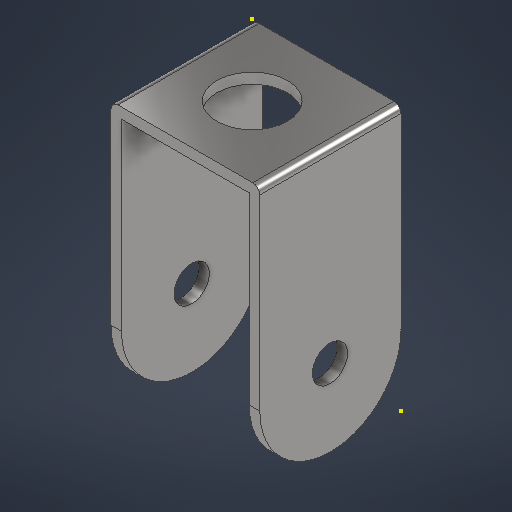
# Autodesk Inventor part: peca1
Saved by Autodesk Inventor 2026 (Build 300175050, 175E)
## iProperties
Created: 2026-05-07
Part Number: peca1
Material: Steel, Carbon
Document SubType Name: Modeling
Designer: Administrator
Density: 7.85 g/cm^3
Appearance: Semi-Polished
Mass: 155.634 g
Surface Area: 148.219 cm^2
Volume: 19.826 cm^3
Author: Administrator
Autodesk Inventor part; units mm, degrees
ref_plane "YZ Plane" through (0, 0, 0) normal (1, 0, 0) x (0, 1, 0)
ref_plane "XZ Plane" through (0, 0, 0) normal (0, 1, 0) x (-1, 0, 0)
ref_plane "XY Plane" through (0, 0, 0) normal (0, 0, 1) x (1, 0, 0)
sketch "Sketch1" plane through (0, 0, 0) normal (0, 0, 1) x (1, 0, 0)
  line L0 (0, 0) -> (3, 0)
  line L1 (3, 0) -> (3, 72)
  line L2 (3, 72) -> (39.1537, 72)
  line L3 (42.1537, 75) -> (0, 75)
  line L4 (0, 75) -> (0, 0)
  line L5 (42.1537, 75) -> (42.1537, 0)
  line L6 (42.1537, 0) -> (39.1537, 0)
  line L7 (39.1537, 0) -> (39.1537, 72)
  dimension "d0" = 75
  dimension "d1" = 3
  dimension "d3" = 3
  constraints: 16 end point, 5 perpendicular, 1 horizontal, 1 vertical
  measures "d0" distance of L3.end L0.start
  measures "d1" distance between parallel lines of L2 L3
  measures "d3" distance between parallel lines of L4 L1
extrude "Extrusion1" add sketch "Sketch1" along normal blind 40
fillet "Fillet1" radius 20 2 edges at (40.6537, 0, 40) (40.6537, 0, 0)
fillet "Fillet2" radius 20 2 edges at (1.5, 0, 40) (1.5, 0, 0)
sketch "Sketch2" plane through (42.1537, 75, 40) normal (1, 0, 0) x (0, 0, -1)
  circle A0 centre (19.8608, -53.2379) radius 5
  point P0 (40, -75)
  dimension "d8" = 10
  constraints: 1 centre point
  measures "d8" diameter of A0
extrude "Extrusion2" cut sketch "Sketch2" against normal blind 50
sketch "Sketch3" plane through (0, 75, 0) normal (0, 1, 0) x (1, 0, 0)
  circle A0 centre (20, -20.0234) radius 10
  line L0 (0, 0) -> (0, -40) projected
  dimension "d11" = 20
  dimension "d12" = 20
  constraints: 1 centre point
  measures "d11" diameter of A0
  measures "d12" distance from line of L0 A0.centre
sketch "Sketch4" plane through (0, 75, 0) normal (0, 1, 0) x (1, 0, 0)
  point P0 (0, 0)
extrude "Extrusion3" cut sketch "Sketch3" against normal through all
fillet "Fillet3" radius 2 2 edges at (42.1537, 75, 20) (0, 75, 20)
sketch "Sketch5" plane through (2, 75, 0) normal (0, 1, 0) x (1, 0, 0)
  point P0 (-2, 0)
sketch "Sketch6" plane through (42.1537, 20, 20) normal (1, 0, 0) x (0, 0, -1)
  point P0 (20, -20)
body "Solid1"
